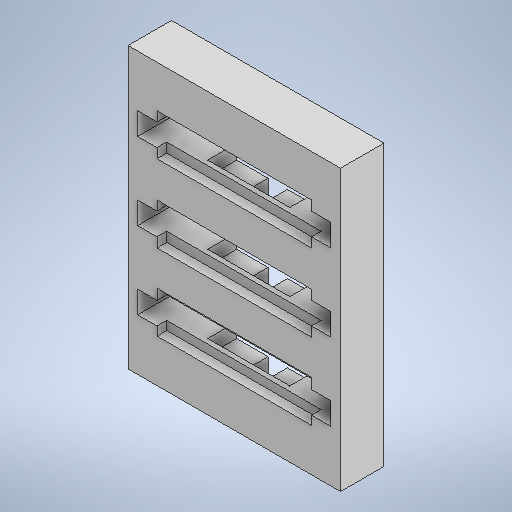
# Autodesk Inventor part: Lightpipe shield
Saved by Autodesk Inventor 2025 (Build 290162000, 162)
## iProperties
Created: 2024-07-18
Part Number: Lightpipe shield
Material: Generic
Document SubType Name: Modeling
Designer: adam
Density: 1 g/cm^3
Appearance: Default
Author: adam
Autodesk Inventor part; units mm, degrees
ref_plane "YZ Plane" through (0, 0, 0) normal (1, 0, 0) x (0, 1, 0)
ref_plane "XZ Plane" through (0, 0, 0) normal (0, 1, 0) x (-1, 0, 0)
ref_plane "XY Plane" through (0, 0, 0) normal (0, 0, 1) x (1, 0, 0)
sketch "Sketch1" plane through (0, 0, 0) normal (0, 0, 1) x (1, 0, 0)
  line L0 (0, 0) -> (22, 0)
  line L1 (22, 0) -> (22, -29)
  line L2 (22, -29) -> (0, -29)
  line L3 (0, -29) -> (0, 0)
  line L4 (3, -5.35) -> (19, -5.35)
  line L5 (19, -5.35) -> (19, -7.65)
  line L6 (19, -7.65) -> (3, -7.65)
  line L7 (3, -7.65) -> (3, -5.35)
  line L8 (3, -13.35) -> (19, -13.35)
  line L9 (19, -13.35) -> (19, -15.65)
  line L10 (19, -15.65) -> (3, -15.65)
  line L11 (3, -15.65) -> (3, -13.35)
  line L12 (3, -21.35) -> (19, -21.35)
  line L13 (19, -21.35) -> (19, -23.65)
  line L14 (19, -23.65) -> (3, -23.65)
  line L15 (3, -23.65) -> (3, -21.35)
  line L16 (19, -5.35) -> (19, -13.35) construction
  line L17 (19, -13.35) -> (19, -21.35) construction
  line L18 (22, -14.5) -> (0, -14.5) construction
  line L19 (11, 0) -> (11, -29) construction
  point P0 (19, -14.5)
  point P1 (11, -5.35)
  dimension "d0" = 22
  dimension "d1" = 29
  dimension "d2" = 2.3
  dimension "d3" = 8
  dimension "d4" = 16
  constraints: 40 end point, 9 point on line, 8 parallel, 6 midpoint, 6 perpendicular, 4 collinear, 4 horizontal
  measures "d0" distance of L0.start L0.end
  measures "d1" distance of L0.end L1.end
  measures "d2" distance of L6.end L4.start
  measures "d3" distance of L16.start L16.end
  measures "d4" distance of L4.start L4.end
extrude "Body with light pipe slots" add sketch "Sketch1" along normal blind 4.5
sketch "Sketch2" plane through (0, 0, 4.5) normal (0, 0, 1) x (1, 0, 0)
  line L0 (0, -29) -> (22, -29) construction
  line L1 (22, -29) -> (22, 0) construction
  line L2 (22, 0) -> (0, 0) construction
  line L3 (0, 0) -> (0, -29) construction
  line L4 (3, -21.35) -> (19, -21.35) construction
  line L5 (19, -21.35) -> (19, -23.65) construction
  line L6 (19, -23.65) -> (3, -23.65) construction
  line L7 (3, -23.65) -> (3, -21.35) construction
  line L8 (3, -13.35) -> (19, -13.35) construction
  line L9 (19, -13.35) -> (19, -15.65) construction
  line L10 (19, -15.65) -> (3, -15.65) construction
  line L11 (3, -15.65) -> (3, -13.35) construction
  line L12 (3, -5.35) -> (19, -5.35) construction
  line L13 (19, -5.35) -> (19, -7.65) construction
  line L14 (19, -7.65) -> (3, -7.65) construction
  line L15 (3, -7.65) -> (3, -5.35) construction
  line L16 (1, -5.35) -> (21, -5.35)
  line L17 (21, -5.35) -> (21, -7.65)
  line L18 (21, -7.65) -> (1, -7.65)
  line L19 (1, -7.65) -> (1, -5.35)
  line L20 (1, -13.35) -> (21, -13.35)
  line L21 (21, -13.35) -> (21, -15.65)
  line L22 (21, -15.65) -> (1, -15.65)
  line L23 (1, -15.65) -> (1, -13.35)
  line L24 (1, -21.35) -> (21, -21.35)
  line L25 (21, -21.35) -> (21, -23.65)
  line L26 (21, -23.65) -> (1, -23.65)
  line L27 (1, -23.65) -> (1, -21.35)
  dimension "d7" = 2
  dimension "d8" = 2
  constraints: 24 end point, 7 point on line, 6 parallel, 3 collinear, 3 horizontal, 3 perpendicular
  measures "d7" distance between parallel lines of L15 L19
  measures "d8" distance between parallel lines of L17 L13
extrude "Light pipe wing cuts" cut sketch "Sketch2" against normal blind 4
sketch "Sketch3" plane through (0, 0, 4.5) normal (0, 0, 1) x (1, 0, 0)
  line L0 (1, -21.35) -> (21, -21.35) construction
  line L1 (21, -21.35) -> (21, -23.65) construction
  line L2 (21, -23.65) -> (1, -23.65) construction
  line L3 (1, -23.65) -> (1, -21.35) construction
  line L4 (1, -13.35) -> (21, -13.35) construction
  line L5 (21, -13.35) -> (21, -15.65) construction
  line L6 (21, -15.65) -> (1, -15.65) construction
  line L7 (1, -15.65) -> (1, -13.35) construction
  line L8 (1, -5.35) -> (21, -5.35) construction
  line L9 (21, -5.35) -> (21, -7.65) construction
  line L10 (21, -7.65) -> (1, -7.65) construction
  line L11 (1, -7.65) -> (1, -5.35) construction
  line L12 (0, -29) -> (22, -29) construction
  line L13 (22, -29) -> (22, 0) construction
  line L14 (22, 0) -> (0, 0) construction
  line L15 (0, 0) -> (0, -29) construction
  line L16 (3, -5.35) -> (3, -7.65) construction
  line L17 (19, -7.65) -> (19, -5.35) construction
  line L18 (19, -15.65) -> (19, -13.35) construction
  line L19 (19, -23.65) -> (19, -21.35) construction
  line L20 (3, -21.35) -> (3, -23.65) construction
  line L21 (3, -13.35) -> (3, -15.65) construction
  line L22 (3, -4.35) -> (19, -4.35)
  line L23 (19, -4.35) -> (19, -8.65)
  line L24 (19, -8.65) -> (3, -8.65)
  line L25 (3, -8.65) -> (3, -4.35)
  line L26 (3, -12.35) -> (19, -12.35)
  line L27 (19, -12.35) -> (19, -16.65)
  line L28 (19, -16.65) -> (3, -16.65)
  line L29 (3, -16.65) -> (3, -12.35)
  line L30 (3, -20.2545) -> (19, -20.2545)
  line L31 (19, -20.2545) -> (19, -24.5545)
  line L32 (19, -24.5545) -> (3, -24.5545)
  line L33 (3, -24.5545) -> (3, -20.2545)
  dimension "d11" = 1
  dimension "d12" = 1
  dimension "d13" = 1.0956
  dimension "d14" = 1
  constraints: 24 end point, 6 parallel, 5 point on line, 3 collinear, 3 horizontal, 3 perpendicular
  measures "d11" distance between parallel lines of L22 L8
  measures "d12" distance between parallel lines of L4 L26
  measures "d13" distance between parallel lines of L30 L0
  measures "d14" distance between parallel lines of L10 L24
extrude "SMD clearance cuts" cut sketch "Sketch3" against normal blind 1
sketch "Sketch4" plane through (0, 0, 0) normal (0, 0, -1) x (-1, 0, 0)
  line L0 (-22, 0) -> (0, 0) construction
  line L1 (-11, 0) -> (-11, -29) construction
  line L2 (0, -29) -> (-22, -29) construction
  line L3 (-12, -2.15) -> (-10, -2.15)
  line L4 (-10, -26.85) -> (-12, -26.85)
  line L5 (-3, -5.35) -> (-19, -5.35) projected
  line L6 (-19, -23.65) -> (-3, -23.65) projected
  line L7 (-6.75, -23.65) -> (-6.75, -25.15)
  line L8 (-15.25, -25.15) -> (-15.25, -23.65)
  line L9 (-19, -15.65) -> (-3, -15.65) projected
  line L10 (-6.75, -15.65) -> (-6.75, -17.15)
  line L11 (-15.25, -17.15) -> (-15.25, -15.65)
  line L12 (-3, -7.65) -> (-19, -7.65) projected
  line L13 (-6.75, -7.65) -> (-6.75, -9.15)
  line L14 (-15.25, -9.15) -> (-15.25, -7.65)
  line L15 (-12, -7.65) -> (-12, -2.15)
  line L16 (-10, -2.15) -> (-10, -7.65)
  line L17 (-6.75, -9.15) -> (-10, -9.15)
  line L18 (-12, -9.15) -> (-15.25, -9.15)
  line L19 (-12, -15.65) -> (-12, -9.15)
  line L20 (-10, -9.15) -> (-10, -15.65)
  line L21 (-15.25, -15.65) -> (-12, -15.65)
  line L22 (-10, -15.65) -> (-6.75, -15.65)
  line L23 (-6.75, -17.15) -> (-10, -17.15)
  line L24 (-12, -17.15) -> (-15.25, -17.15)
  line L25 (-15.25, -23.65) -> (-12, -23.65)
  line L26 (-10, -23.65) -> (-6.75, -23.65)
  line L27 (-6.75, -25.15) -> (-10, -25.15)
  line L28 (-12, -25.15) -> (-15.25, -25.15)
  line L29 (-12, -26.85) -> (-12, -25.15)
  line L30 (-12, -23.65) -> (-12, -17.15)
  line L31 (-10, -17.15) -> (-10, -23.65)
  line L32 (-10, -25.15) -> (-10, -26.85)
  line L33 (-15.25, -7.65) -> (-12, -7.65)
  line L34 (-10, -7.65) -> (-6.75, -7.65)
  point P0 (-11, -2.15)
  dimension "d17" = 3.2
  dimension "d18" = 2
  dimension "d19" = 3.2
  dimension "d20" = 1.5
  dimension "d21" = 8.5
  dimension "d22" = 4.25
  constraints: 58 end point, 32 parallel, 10 perpendicular, 8 point on line, 7 horizontal, 5 equal length, 3 collinear, 3 midpoint
  measures "d17" distance between parallel lines of L5 L3
  measures "d18" distance of L3.start L3.end
  measures "d19" distance between parallel lines of L6 L4
  measures "d20" distance of L14.start L14.end
  measures "d21" distance of L13.end L14.start
  measures "d22" distance between parallel lines of L1 L14
extrude "Case interior molding cuts" cut sketch "Sketch4" against normal blind 3
equation "\"d8\" = d7"
equation "\"d12\" = d11"
equation "\"d14\" = d11"
equation "\"d22\" = 0.5 * d21"
body "Solid1"
